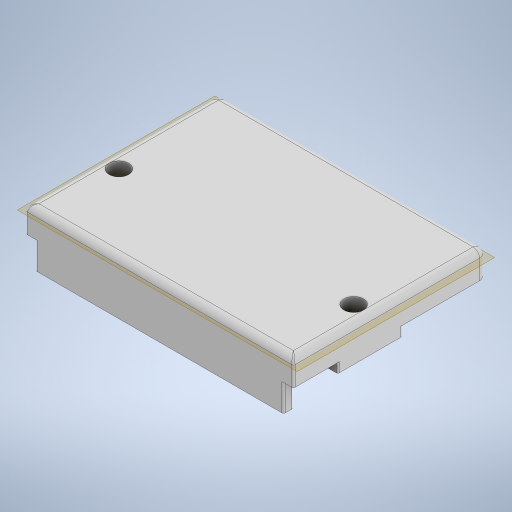
# Autodesk Inventor part: dach
Saved by Autodesk Inventor 2023 (Build 270158000, 158)
## iProperties
Created: 2024-04-28
Part Number: dach
Material: Ogólny
Document SubType Name: Modeling
Designer: kamil
Density: 1 g/cm^3
Appearance: Domyślna
Author: kamil
Autodesk Inventor part; units mm, degrees
ref_plane "YZ Plane" through (0, 0, 0) normal (1, 0, 0) x (0, 1, 0)
ref_plane "XZ Plane" through (0, 0, 0) normal (0, 1, 0) x (-1, 0, 0)
ref_plane "XY Plane" through (0, 0, 0) normal (0, 0, 1) x (1, 0, 0)
sketch "Szkic1" plane through (0, 0, 0) normal (0, 1, 0) x (-1, 0, 0)
  line L0 (41, 29.5365) -> (-41, 29.5365)
  line L1 (-41, 29.5365) -> (-41, -29.5365)
  line L2 (-41, -29.5365) -> (41, -29.5365)
  line L3 (41, -29.5365) -> (41, 29.5365)
  point P0 (0, 0)
  point P1 (41, 0)
  point P2 (0, -29.5365)
  dimension "d0" = 82
  dimension "d1" = 59.073
  constraints: 8 end point, 2 midpoint, 2 parallel, 1 horizontal, 1 horizontal alignment, 1 perpendicular, 1 vertical alignment
  measures "d0" distance of L1.end L2.end
  measures "d1" distance of L2.end L0.start
extrude "Wyciągnięcie proste1" add sketch "Szkic1" along normal blind 8
sketch "Szkic2" plane through (0, 0, 0) normal (0, -1, 0) x (1, 0, 0)
  line L0 (41, 29.5365) -> (41, -29.5365) projected
  line L1 (-41, 29.5365) -> (41, 29.5365) projected
  line L2 (-41, -29.5365) -> (-41, 29.5365) projected
  line L3 (41, -29.5365) -> (-41, -29.5365) projected
  line L4 (41, 29.5365) -> (41, -29.5365) projected
  line L5 (41, 29.5365) -> (38.1, 29.5365)
  line L6 (38.1, 29.5365) -> (38.1, 15.9365)
  line L7 (38.1, 15.9365) -> (41, 15.9365)
  line L8 (41, 15.9365) -> (41, 29.5365)
  line L9 (-41, -29.5365) -> (-41, 29.5365) projected
  line L10 (-41, 29.5365) -> (-38.1, 29.5365)
  line L11 (-38.1, 29.5365) -> (-38.1, 15.9365)
  line L12 (-38.1, 15.9365) -> (-41, 15.9365)
  line L13 (-41, 15.9365) -> (-41, 29.5365)
  line L14 (41, 15.9365) -> (31, 15.9365)
  line L15 (31, 15.9365) -> (31, -3.8635)
  line L16 (31, -3.8635) -> (41, -3.8635)
  line L17 (41, -3.8635) -> (41, 15.9365)
  line L18 (-41, 15.9365) -> (-31, 15.9365)
  line L19 (-31, 15.9365) -> (-31, -3.8635)
  line L20 (-31, -3.8635) -> (-41, -3.8635)
  line L21 (-41, -3.8635) -> (-41, 15.9365)
  line L22 (41, -29.5365) -> (-41, -29.5365) projected
  line L23 (41, -3.8635) -> (38.1, -3.8635)
  line L24 (38.1, -3.8635) -> (38.1, -29.5365)
  line L25 (38.1, -29.5365) -> (41, -29.5365)
  line L26 (41, -29.5365) -> (41, -3.8635)
  line L27 (-41, -3.8635) -> (-38.1, -3.8635)
  line L28 (-38.1, -3.8635) -> (-38.1, -29.5365)
  line L29 (-38.1, -29.5365) -> (-41, -29.5365)
  line L30 (-41, -29.5365) -> (-41, -3.8635)
  line L31 (-41, -29.5365) -> (-27.25, -29.5365)
  line L32 (-27.25, -29.5365) -> (-27.25, -26.6365)
  line L33 (-27.25, -26.6365) -> (-41, -26.6365)
  line L34 (-41, -26.6365) -> (-41, -29.5365)
  line L35 (41, -29.5365) -> (27.25, -29.5365)
  line L36 (27.25, -29.5365) -> (27.25, -26.6365)
  line L37 (27.25, -26.6365) -> (41, -26.6365)
  line L38 (41, -26.6365) -> (41, -29.5365)
  line L39 (27.25, -29.5365) -> (-27.25, -29.5365)
  line L40 (-27.25, -29.5365) -> (-27.25, -19.5365)
  line L41 (-27.25, -19.5365) -> (27.25, -19.5365)
  line L42 (27.25, -19.5365) -> (27.25, -29.5365)
  point P0 (0, 0)
  point P1 (-27.25, -24.5365)
  point P2 (0, -19.5365)
  point P3 (-41, 15.9365)
  point P4 (-41, -3.8635)
  dimension "d4" = 2.9
  dimension "d6" = 2.9
  dimension "d7" = 10
  dimension "d8" = 19.8
  dimension "d9" = 10
  dimension "d10" = 2.9
  dimension "d11" = 2.9
  dimension "d13" = 2.9
  dimension "d17" = 10
  dimension "d18" = 19.8
  dimension "d19" = 54.5
  dimension "d32" = 13.6
  dimension "d33" = 13.6
  constraints: 72 end point, 18 parallel, 9 horizontal, 9 perpendicular, 3 point on line, 2 midpoint, 2 vertical alignment
  measures "d4" distance of L7.end L6.end
  measures "d6" distance of L11.end L12.end
  measures "d7" distance of L16.end L15.end
  measures "d8" distance of L14.end L15.end
  measures "d9" distance of L19.end L20.end
  measures "d10" distance of L25.end L24.end
  measures "d11" distance of L28.end L29.end
  measures "d13" distance of L32.end L31.end
  measures "d17" distance of L39.end L40.end
  measures "d18" distance of L18.end L19.end
  measures "d19" distance of L40.end L41.end
  measures "d32" distance between parallel lines of L1 L14
  measures "d33" distance between parallel lines of L1 L18
extrude "Wyciągnięcie proste2" add sketch "Szkic2" along normal blind 2.95 contours L0 L16 L15 L14 L7 | L18 L19 L20 L2 L12
fillet "Zaokrąglenie1" radius 6 4 edges at (31, -1.475, 15.9365) (31, -1.475, -3.8635) (-31, -1.475, -3.8635) (-31, -1.475, 15.9365)
fillet "Zaokrąglenie2" radius 2 2 edges at (41, 4, -29.5365) (-41, 4, -29.5365)
sketch "Szkic3" plane through (0, 0, 0) normal (0, -1, 0) x (1, 0, 0)
  line L0 (41, 29.5365) -> (41, 15.9365) projected
  line L1 (-41, 29.5365) -> (41, 29.5365) projected
  line L2 (-41, 15.9365) -> (-41, 29.5365) projected
  line L3 (38, 26.6365) -> (-38, 26.6365)
  line L4 (-38, 26.6365) -> (-38, 29.5365)
  line L5 (-38, 29.5365) -> (38, 29.5365)
  line L6 (38, 29.5365) -> (38, 26.6365)
  point P0 (0, 0)
  point P1 (0, 26.6365)
  point P2 (0, 29.5365)
  point P3 (0, 29.5365)
  point P4 (0, 29.5365)
  dimension "d24" = 76
  dimension "d25" = 2.9
  constraints: 8 end point, 4 midpoint, 2 parallel, 1 coincident, 1 horizontal, 1 perpendicular, 1 vertical alignment
  measures "d24" distance of L4.end L5.end
  measures "d25" distance of L3.end L4.end
extrude "Wyciągnięcie proste3" add sketch "Szkic3" along normal blind 8.3
fillet "Zaokrąglenie5" radius 0.5 2 edges at (-41, 4, 29.5365) (41, 4, 29.5365)
sketch "Szkic4" plane through (0, 8, 0) normal (0, 1, 0) x (1, 0, 0)
  arc A0 (-37, -15.9365) -> (-31, -9.9365) centre (-37, -9.9365) ccw projected
  line L0 (-37, -15.9365) -> (-41, -15.9365) projected
  line L1 (-41, -15.9365) -> (-41, 3.8635) projected
  line L2 (-41, 3.8635) -> (-37, 3.8635) projected
  arc A1 (-31, -2.1365) -> (-37, 3.8635) centre (-37, -2.1365) ccw projected
  line L3 (-31, -2.1365) -> (-31, -9.9365) projected
  arc A2 (37, 3.8635) -> (31, -2.1365) centre (37, -2.1365) ccw projected
  line L4 (37, 3.8635) -> (41, 3.8635) projected
  line L5 (41, 3.8635) -> (41, -15.9365) projected
  line L6 (41, -15.9365) -> (37, -15.9365) projected
  arc A3 (31, -9.9365) -> (37, -15.9365) centre (37, -9.9365) ccw projected
  line L7 (31, -9.9365) -> (31, -2.1365) projected
  line L8 (-31, -6.0365) -> (-41, -6.0365) construction
  line L9 (41, -6.0365) -> (31, -6.0365) construction
  point P0 (0, 0)
  point P1 (36, -6.0365)
  point P2 (-36, -6.0365)
  point P3 (36, -6.0365)
  point P4 (-36, -6.0365)
  constraints: 6 midpoint, 4 coincident, 4 end point
hole "Otwór1" at (36, 8, 6.0365) at (-36, 8, 6.0365) direction (0, -1, 0) diameter 3.2 end through all counterbore diameter 6 counterbore depth 4
fillet "Zaokrąglenie7" radius 2 8 edges at (40.4142, 8, -28.9507) (0, 8, -29.5365) (-40.4142, 8, -28.9507) (-41, 8, 0.75) (-40.8536, 8, 29.3901) (0, 8, 29.5365) (40.8536, 8, 29.3901) (41, 8, 0.75)
ref_plane "Płaszczyzna konstrukcyjna1" through (0, 5.75, 0) normal (0, 1, 0) x (1, 0, 0)
sketch "Szkic5" plane through (0, 5.75, 0) normal (0, 1, 0) x (1, 0, 0)
  line L0 (0, 41.3519) -> (0, -41.3557) projected
  line L1 (57.4054, 0) -> (-57.4054, 0) projected
  line L2 (38, -29.5365) -> (-38, -29.5365) projected
  point P0 (0, 0)
  point P1 (0, -17.5365)
  point P2 (-12, -17.5365)
  point P3 (-24, -17.5365)
  point P4 (0, -5.5365)
  point P5 (-12, -5.5365)
  point P6 (-24, -5.5365)
  point P7 (0, 6.4635)
  point P8 (-12, 6.4635)
  point P9 (-24, 6.4635)
  point P10 (0, 18.4635)
  point P11 (-12, 18.4635)
  point P12 (-24, 18.4635)
  point P13 (12, -17.5365)
  point P14 (24, -17.5365)
  point P15 (0, -5.5365)
  point P16 (12, -5.5365)
  point P17 (24, -5.5365)
  point P18 (0, 6.4635)
  point P19 (12, 6.4635)
  point P20 (24, 6.4635)
  point P21 (0, 18.4635)
  point P22 (12, 18.4635)
  point P23 (24, 18.4635)
  dimension "d43" = 12
  dimension "d46" = 12
  dimension "d49" = 12
  dimension "d54" = 12
  dimension "d57" = 12
  constraints: 2 horizontal, 2 vertical, 1 point on line, 22 other
  measures "d43" distance from line of L2 point (0, -17.536)
  measures "d46" distance of point (0, -17.536) point (-12, -17.536)
  measures "d49" distance of point (0, -17.536) point (0, -5.536)
  measures "d54" distance of point (0, -17.536) point (12, -17.536)
  measures "d57" distance of point (0, -17.536) point (0, -5.536)
hole "Otwór2" at (0, 5.75, 17.5365) at (-12, 5.75, 17.5365) at (-24, 5.75, 17.5365) at (0, 5.75, 5.5365) at (-12, 5.75, 5.5365) at (-24, 5.75, 5.5365) at (0, 5.75, -6.4635) at (-12, 5.75, -6.4635) at (-24, 5.75, -6.4635) at (0, 5.75, -18.4635) at (-12, 5.75, -18.4635) at (-24, 5.75, -18.4635) at (12, 5.75, 17.5365) at (24, 5.75, 17.5365) at (12, 5.75, 5.5365) at (24, 5.75, 5.5365) at (12, 5.75, -6.4635) at (24, 5.75, -6.4635) at (12, 5.75, -18.4635) at (24, 5.75, -18.4635) direction (0, -1, 0) diameter 5.5 depth 3.5
fillet "Zaokrąglenie10" radius 2 1 edges at (0, 0, 26.6365)
fillet "Zaokrąglenie11" radius 0.5 10 edges at (38, -0.5858, 26.0507) (38, -5.15, 26.6365) (38, -4.15, 29.5365) (-38, -0.5858, 26.0507) (-38, -5.15, 26.6365) (-38, -4.15, 29.5365) (-41, -1.475, -3.8635) (-41, -1.475, 15.9365) (41, -1.475, -3.8635) (41, -1.475, 15.9365)
